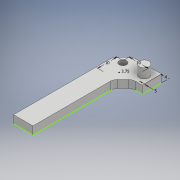
# Autodesk Inventor part: garabber2
Saved by Autodesk Inventor 2018.2 (Build 222227000, 227)
## iProperties
Created: 2018-03-18
Part Number: garabber2
Material: Generic
Document SubType Name: Modeling
Designer: mzhang
Density: 1 g/cm^3
Appearance: Default
Author: mzhang
Autodesk Inventor part; units mm, degrees
ref_plane "YZ Plane" through (0, 0, 0) normal (1, 0, 0) x (0, 1, 0)
ref_plane "XZ Plane" through (0, 0, 0) normal (0, 1, 0) x (-1, 0, 0)
ref_plane "XY Plane" through (0, 0, 0) normal (0, 0, 1) x (1, 0, 0)
sketch "Sketch1" plane through (0, 0, 0) normal (0, 0, 1) x (1, 0, 0)
  circle A0 centre (0, 0) radius 1.875
  line L0 (5, -5) -> (-5, -5)
  line L1 (-5, -5) -> (-5, 5)
  line L2 (-5, 5) -> (5, 5)
  line L3 (5, 5) -> (5, -5)
  line L4 (5, -5) -> (-5, 5) construction
  line L5 (-5, -5) -> (5, 5) construction
  line L6 (-5, -5) -> (5, -5)
  line L7 (5, -5) -> (5, -51.5367)
  line L8 (5, -51.5367) -> (-5, -51.5367)
  line L9 (-5, -51.5367) -> (-5, -5)
  line L10 (5, 5) -> (15, 5)
  line L11 (15, 5) -> (15, -5)
  line L12 (15, -5) -> (5, -5)
  line L13 (5, -5) -> (5, 5)
  circle A1 centre (11, 0) radius 2.5
  dimension "d0" = 3.75
  dimension "d1" = 10
  dimension "d2" = 10
  dimension "d3" = 5
  dimension "d4" = 4
  constraints: 28 end point, 6 parallel, 3 horizontal, 3 perpendicular, 2 centre point, 2 midpoint, 1 coincident
  measures "d0" diameter of A0
  measures "d1" distance of L1.end L2.end
  measures "d2" distance of L0.end L1.end
  measures "d3" diameter of A1
  measures "d4" distance from line of L11 A1.centre
extrude "Extrusion1" add sketch "Sketch1" along normal blind 4
chamfer "Chamfer1" distance 5 angle 45 1 edges at (5, -5, 2)
extrude "Extrusion2" add sketch "Sketch1" along normal blind 9 contours A1
chamfer "Chamfer2" distance 5 angle 45 1 edges at (-5, 5, 2)
fillet "Fillet1" radius 4 2 edges at (0, 5, 2) (-5, 0, 2)
fillet "Fillet2" radius 4 2 edges at (5, -10, 2) (10, -5, 2)
body "Solid1"
